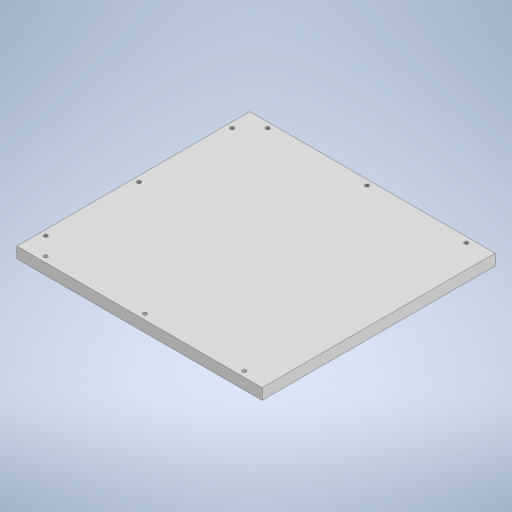
# Autodesk Inventor part: BaseEmbaixoFuros
Saved by Autodesk Inventor 2023.2 (Build 272271030, 271C)
## iProperties
Created: 2023-04-15
Part Number: BaseEmbaixoFuros
Material: Generic
Document SubType Name: Modeling
Designer: victo
Density: 1 g/cm^3
Appearance: Default
Author: victo
## iProperties of the stored document BaseEncima_3DPrint.ipt
Created: 2023-05-16
Part Number: BaseEncima_3DPrint
Material: Generic
Document SubType Name: Modeling
Designer: VICTOR
Density: 1 g/cm^3
Appearance: Default
Author: VICTOR
Autodesk Inventor part; units mm, degrees
ref_plane "YZ Plane" through (0, 0, 0) normal (1, 0, 0) x (0, 1, 0)
ref_plane "XZ Plane" through (0, 0, 0) normal (0, 1, 0) x (-1, 0, 0)
ref_plane "XY Plane" through (0, 0, 0) normal (0, 0, 1) x (1, 0, 0)
sketch "Sketch1" plane through (0, 0, 0) normal (0, 1, 0) x (-1, 0, 0)
  line L0 (0, 0) -> (200, 0)
  line L1 (200, 0) -> (200, -190)
  line L2 (200, -190) -> (0, -190)
  line L3 (0, -190) -> (0, 0)
  dimension "d0" = 200
  dimension "d1" = 190
  constraints: 8 end point, 2 parallel, 1 horizontal, 1 perpendicular
  measures "d0" distance of L1.end L2.end
  measures "d1" distance of L0.end L1.end
extrude "Extrusion1" add sketch "Sketch1" along normal blind 9
sketch "Sketch14" plane through (0, 9, 0) normal (0, 1, 0) x (1, 0, 0)
  line L0 (0, 190) -> (-200, 190) projected
  line L1 (-200, 190) -> (-200, 0) projected
  line L2 (-200, 0) -> (0, 0) projected
  line L3 (0, 0) -> (0, 190) projected
  line L4 (-200, 190) -> (-200, 0) projected
  line L5 (-200, 190) -> (0, 190)
  line L6 (0, 190) -> (0, 181)
  line L7 (0, 181) -> (-200, 181)
  line L8 (-200, 181) -> (-200, 190)
  line L9 (-200, 0) -> (0, 0) projected
  line L10 (-200, 181) -> (-191, 181)
  line L11 (-191, 181) -> (-191, 0)
  line L12 (-191, 0) -> (-200, 0)
  line L13 (-200, 0) -> (-200, 181)
  line L14 (0, 0) -> (0, 190) projected
  line L15 (-191, 0) -> (0, 0)
  line L16 (0, 0) -> (0, 9)
  line L17 (0, 9) -> (-191, 9)
  line L18 (-191, 9) -> (-191, 0)
  circle A0 centre (-19, 4.5) radius 1.5
  circle A1 centre (-100, 4.5) radius 1.5
  circle A2 centre (-181, 4.5) radius 1.5
  line L19 (-245.0017, 95) -> (56.9583, 95)
  circle A3 centre (-19, 185.5) radius 1.5
  circle A4 centre (-100, 185.5) radius 1.5
  circle A5 centre (-181, 185.5) radius 1.5
  circle A6 centre (-195.5, 95) radius 1.5
  circle A7 centre (-195.5, 171) radius 1.5
  circle A8 centre (-195.5, 19) radius 1.5
  dimension "d47" = 9
  dimension "d48" = 9
  dimension "d49" = 9
  dimension "d50" = 3
  dimension "d51" = 3
  dimension "d52" = 3
  dimension "d55" = 3
  dimension "d56" = 3
  dimension "d57" = 3
  dimension "d60" = 19
  constraints: 26 end point, 9 centre point, 6 parallel, 4 horizontal, 4 point on line, 3 perpendicular, 3 symmetric about line, 3 other
  measures "d47" distance of L5.end L6.end
  measures "d48" distance of L11.end L12.end
  measures "d49" distance of L16.end L15.end
  measures "d50" diameter of A0
  measures "d51" diameter of A1
  measures "d52" diameter of A2
  measures "d55" diameter of A6
  measures "d56" diameter of A7
  measures "d57" diameter of A8
  measures "d60" distance from line of L3 A0.centre
extrude "Extrusion14" cut sketch "Sketch14" against normal blind 10 contours A0 | A1 | A2 | A3 | A4 | A5
extrude "Extrusion15" cut sketch "Sketch14" against normal blind 10 contours A6 L19 | L19 A6 | A7 | A8
body "Solid1"
